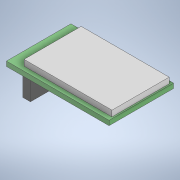
# Autodesk Inventor part: PCB-AE-AQM0802
Saved by Autodesk Inventor 2022 (Build 260153000, 153)
## iProperties
Created: 2024-07-03
Part Number: PCB-AE-AQM0802
Material: 一般
Document SubType Name: Modeling
Designer: yamashita1
Density: 1 g/cm^3
Appearance: 既定
Author: yamashita1
Autodesk Inventor part; units mm, degrees
ref_plane "YZ Plane" through (0, 0, 0) normal (1, 0, 0) x (0, 1, 0)
ref_plane "XZ Plane" through (0, 0, 0) normal (0, 1, 0) x (-1, 0, 0)
ref_plane "XY Plane" through (0, 0, 0) normal (0, 0, 1) x (1, 0, 0)
sketch "スケッチ1" plane through (0, 0, 0) normal (0, 0, 1) x (1, 0, 0)
  line L0 (-17.5, 11) -> (17.5, 11)
  line L1 (17.5, 11) -> (17.5, -11)
  line L2 (17.5, -11) -> (-17.5, -11)
  line L3 (-17.5, -11) -> (-17.5, 11)
  point P0 (0, 0)
  point P1 (-17.5, 0)
  point P2 (0, 11)
  dimension "d0" = 35
  dimension "d1" = 22
  constraints: 8 end point, 2 midpoint, 2 parallel, 1 horizontal, 1 horizontal alignment, 1 perpendicular, 1 vertical alignment
  measures "d0" distance of L1.end L2.end
  measures "d1" distance of L0.end L1.end
extrude "押し出し1" add sketch "スケッチ1" along normal blind 1.6
sketch "スケッチ2" plane through (0, 0, 0) normal (0, 0, -1) x (-1, 0, 0)
  line L0 (15.24, 13.4783) -> (15.24, -13.8825) construction
  line L1 (17.5, 11) -> (17.5, -11) construction
  line L2 (18.6717, -5.08) -> (13.4177, -5.08) construction
  line L3 (17.5, -11) -> (-17.5, -11) construction
  line L4 (13.97, -6.35) -> (16.51, -6.35)
  line L5 (16.51, -6.35) -> (16.51, 6.35)
  line L6 (16.51, 6.35) -> (13.97, 6.35)
  line L7 (13.97, 6.35) -> (13.97, -6.35)
  point P0 (0, 0)
  point P1 (15.24, -6.35)
  dimension "d4" = 2.26
  dimension "d5" = 5.92
  dimension "d6" = 2.54
  dimension "d7" = 1.27
  dimension "d8" = 12.7
  constraints: 12 end point, 2 horizontal, 2 parallel, 1 midpoint, 1 perpendicular, 1 point on line, 1 vertical
  measures "d4" distance between parallel lines of L1 L0
  measures "d5" distance between parallel lines of L3 L2
  measures "d6" distance of L6.end L5.end
  measures "d7" distance between parallel lines of L2 L4
  measures "d8" distance of L4.end L5.end
extrude "押し出し2" add sketch "スケッチ2" along normal blind 11
sketch "スケッチ3" plane through (0, 0, 1.6) normal (0, 0, 1) x (1, 0, 0)
  line L0 (-13, 10) -> (17, 10)
  line L1 (17, 10) -> (17, -9.5)
  line L2 (17, -9.5) -> (-13, -9.5)
  line L3 (-13, -9.5) -> (-13, 10)
  line L4 (17.5, 11) -> (-17.5, 11) projected
  line L5 (17.5, -11) -> (17.5, 11) projected
  point P0 (0, 0)
  dimension "d11" = 30
  dimension "d12" = 19.5
  dimension "d13" = 1
  dimension "d14" = 0.5
  constraints: 8 end point, 2 parallel, 1 horizontal, 1 perpendicular
  measures "d11" distance of L1.end L2.end
  measures "d12" distance of L0.end L1.end
  measures "d13" distance between parallel lines of L4 L0
  measures "d14" distance between parallel lines of L5 L1
extrude "押し出し3" add sketch "スケッチ3" along normal blind 2
